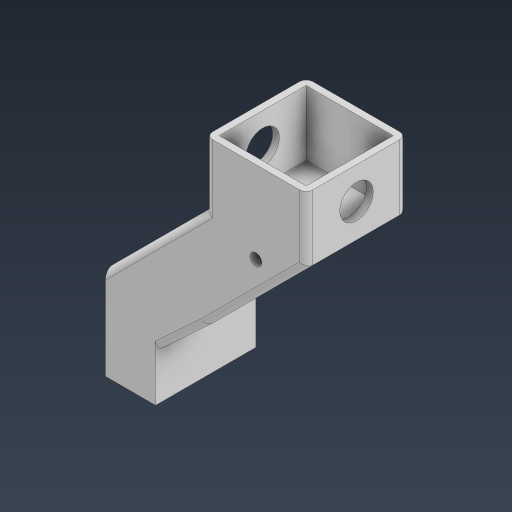
# Autodesk Inventor part: Arm
Saved by Autodesk Inventor 2024 (Build 280153000, 153)
## iProperties
Created: 2023-12-28
Part Number: Arm
Material: Generic
Document SubType Name: Modeling
Designer: Piter
Density: 1 g/cm^3
Appearance: Default
Author: Piter
Autodesk Inventor part; units mm, degrees
ref_plane "YZ Plane" through (0, 0, 0) normal (1, 0, 0) x (0, 1, 0)
ref_plane "XZ Plane" through (0, 0, 0) normal (0, 1, 0) x (-1, 0, 0)
ref_plane "XY Plane" through (0, 0, 0) normal (0, 0, 1) x (1, 0, 0)
sketch "Sketch1" plane through (0, 0, 0) normal (0, 0, 1) x (1, 0, 0)
  line L0 (0, 0) -> (30, 0)
  line L1 (30, 0) -> (30, 20)
  line L2 (30, 20) -> (0, 20)
  line L3 (0, 20) -> (0, 0)
  line L4 (0, 0) -> (-30, 0)
  line L5 (-30, 0) -> (-30, -30)
  line L6 (-30, -30) -> (0, 0)
  line L7 (30, 0) -> (0, -30)
  line L8 (0, -30) -> (-30, -30)
  line L9 (0, -30) -> (-30, -57.7609)
  line L10 (-30, -57.7609) -> (-30, -30)
  line L11 (-30, -15) -> (-15, -15)
  line L12 (-30, -43.8805) -> (-15, -43.8805)
  line L13 (-15, -43.8805) -> (-15, -57.7609)
  line L14 (-15, -57.7609) -> (-30, -57.7609)
  dimension "d0" = 30
  dimension "d1" = 20
  dimension "d2" = 30
  dimension "d3" = 30
  constraints: 30 end point, 5 perpendicular, 4 midpoint, 3 parallel, 2 horizontal, 1 point on line, 1 vertical
  measures "d0" distance of L2.end L1.end
  measures "d1" distance of L1.end L0.end
  measures "d2" distance of L0.start L4.end
  measures "d3" distance of L4.end L5.end
extrude "Extrusion1" add sketch "Sketch1" along normal blind 30 contours L3 L2 L1 L0 | L0 L7 L8 L6 | L9 L12 L10 L8 | L13 L14 L9 | L9 L10 L12
sketch "Sketch2" plane through (0, 20, 0) normal (0, 1, 0) x (1, 0, 0)
  line L0 (30, 0) -> (0, 0) projected
  line L1 (30, -30) -> (0, -30) projected
  line L2 (30, 0) -> (0, 0)
  line L3 (0, 0) -> (0, -30)
  line L4 (0, -30) -> (30, -30)
  line L5 (30, -30) -> (30, 0)
  line L6 (28, -2) -> (2, -2)
  line L7 (2, -2) -> (2, -28)
  line L8 (2, -28) -> (28, -28)
  line L9 (28, -28) -> (28, -2)
  dimension "d6" = 2
  constraints: 16 end point, 4 parallel, 2 perpendicular, 1 horizontal, 3 other
  measures "d6" distance between parallel lines of L5 L9
extrude "Extrusion2" cut sketch "Sketch2" against normal blind 20 contours L9 L8 L7 L6
sketch "Sketch3" plane through (0, 0, 0) normal (-1, 0, 0) x (0, 0, 1)
  line L0 (0, 20) -> (0, 0) projected
  line L1 (0, 10) -> (30, 10)
  line L2 (30, 20) -> (30, 0) projected
  circle A0 centre (15, 10) radius 5
  dimension "d9" = 10
  constraints: 3 midpoint, 2 end point, 1 centre point
  measures "d9" diameter of A0
extrude "Extrusion3" cut sketch "Sketch3" against normal through all
fillet "Fillet1" radius 2 10 edges at (-15, -15, 0) (0, 10, 0) (-15, -15, 30) (0, 10, 30) (15, -15, 30) (30, 10, 30) (15, -15, 0) (30, 10, 0) (-7.5, -36.9402, 0) (-7.5, -36.9402, 30)
sketch "Sketch4" plane through (0, 0, 30) normal (0, 0, 1) x (1, 0, 0)
  line L0 (2, 20) -> (28, 20) projected
  line L1 (15, 20) -> (15, -5)
  circle A0 centre (15, -5) radius 1.75
  point P0 (0, 0)
  dimension "d13" = 25
  dimension "d14" = 3.5
  constraints: 2 end point, 1 centre point, 1 coincident, 1 midpoint, 1 vertical
  measures "d13" distance of L1.start L1.end
  measures "d14" diameter of A0
extrude "Extrusion4" cut sketch "Sketch4" against normal blind 30
move faces "Move1" translate (0, -0.5, 0) faces at (1.3333, 20, 10.6667)
body "Solid1"
